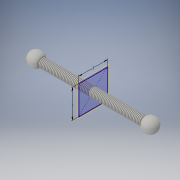
# Autodesk Inventor part: crossbar
Saved by Autodesk Inventor 2016 (Build 200138000, 138)
## iProperties
Created: 2016-04-21
Part Number: crossbar
Material: Generic
Document SubType Name: Modeling
Designer: Sam
Density: 1 g/cm^3
Appearance: Default
Author: Sam
Autodesk Inventor part; units mm, degrees
ref_plane "YZ Plane" through (0, 0, 0) normal (1, 0, 0) x (0, 1, 0)
ref_plane "XZ Plane" through (0, 0, 0) normal (0, 1, 0) x (-1, 0, 0)
ref_plane "XY Plane" through (0, 0, 0) normal (0, 0, 1) x (1, 0, 0)
sketch "Sketch1" plane through (0, 0, 0) normal (1, 0, 0) x (0, 1, 0)
  circle A0 centre (0, 0) radius 1.5
  dimension "d0" = 3
  constraints: 1 centre point, 1 coincident
  measures "d0" diameter of A0
extrude "Extrusion1" add sketch "Sketch1" along normal mid plane 40
sketch "Sketch2" plane through (0, 0, 0) normal (0, 1, 0) x (-1, 0, 0)
  line L0 (20, -1.5) -> (20, 1.5) projected
  arc A0 (17.5, 0) -> (22.5, 0) centre (20, 0) ccw
  line L1 (-20, 1.5) -> (-20, -1.5) projected
  arc A1 (-22.5, 0) -> (-17.5, 0) centre (-20, 0) ccw
  line L2 (22.5, 0) -> (17.5, 0)
  line L3 (-17.5, 0) -> (-22.5, 0)
  line L4 (28.1504, 0) -> (39.5564, 0) construction
  point P0 (0, 0)
  dimension "d3" = 5
  dimension "d4" = 5
  constraints: 6 end point, 4 point on circle, 3 horizontal, 2 centre point, 2 midpoint
  measures "d3" diameter of A0
  measures "d4" diameter of A1
revolve "Revolution1" add sketch "Sketch2" angle 360 about axis through (-28.1504, 0, 0) along (-1, 0, 0)
thread "Thread1" size "M3x0.5" class "6g" standard "ANSI Metric M Profile" full length
sketch "Sketch3" plane through (0, 0, 0) normal (1, 0, 0) x (0, 1, 0)
  line L0 (-5, -5) -> (5, -5)
  line L1 (5, -5) -> (5, 5)
  line L2 (5, 5) -> (-5, 5)
  line L3 (-5, 5) -> (-5, -5)
  line L4 (-5, -5) -> (5, 5) construction
  line L5 (5, -5) -> (-5, 5) construction
  point P0 (0, 0)
  dimension "d8" = 10
  dimension "d9" = 10
  constraints: 12 end point, 2 midpoint, 2 parallel, 1 horizontal, 1 perpendicular
  measures "d8" distance of L2.end L1.end
  measures "d9" distance of L1.end L0.end
ref_plane "Work Plane1" through (0, 5, -5) normal (-1, 0, 0) x (0, 0, 1)
body "Solid1"
